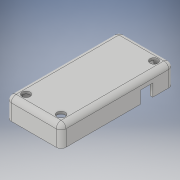
# Autodesk Inventor part: Topcase
Saved by Autodesk Inventor 2019 (Build 230136000, 136)
## iProperties
Created: 2019-05-05
Part Number: Topcase
Material: Generic
Document SubType Name: Modeling
Designer: Henry
Density: 1 g/cm^3
Appearance: Default
Author: Henry
Autodesk Inventor part; units mm, degrees
ref_plane "YZ Plane" through (0, 0, 0) normal (1, 0, 0) x (0, 1, 0)
ref_plane "XZ Plane" through (0, 0, 0) normal (0, 1, 0) x (-1, 0, 0)
ref_plane "XY Plane" through (0, 0, 0) normal (0, 0, 1) x (1, 0, 0)
sketch "Sketch1" plane through (0, 0, 0) normal (0, 1, 0) x (-1, 0, 0)
  line L0 (0, 0) -> (40.5, 0)
  line L1 (40.5, 0) -> (40.5, -87.5)
  line L2 (40.5, -87.5) -> (0, -87.5)
  line L3 (0, -87.5) -> (0, 0)
  dimension "d0" = 40.5
  dimension "d1" = 87.5
  constraints: 8 end point, 2 parallel, 1 horizontal, 1 perpendicular
  measures "d0" distance of L1.end L2.end
  measures "d1" distance of L0.end L1.end
extrude "Extrusion1" add sketch "Sketch1" along normal blind 2
sketch "Sketch4" plane through (0, 2, 0) normal (0, 1, 0) x (1, 0, 0)
  line L0 (0, 0) -> (2, 0)
  line L1 (2, 0) -> (2, 87.5)
  line L2 (2, 87.5) -> (0, 87.5)
  line L3 (0, 87.5) -> (0, 0)
  line L4 (-40.5, 87.5) -> (-40.5, 0) projected
  line L5 (-40.5, 0) -> (-42.5, 0)
  line L6 (-42.5, 0) -> (-42.5, 87.5)
  line L7 (-42.5, 87.5) -> (-40.5, 87.5)
  line L8 (-40.5, 87.5) -> (-40.5, 0)
  line L9 (-42.5, 0) -> (2, 0)
  line L10 (2, 0) -> (2, -2)
  line L11 (2, -2) -> (-42.5, -2)
  line L12 (-42.5, -2) -> (-42.5, 0)
  line L13 (2, 87.5) -> (-42.5, 87.5)
  line L14 (-42.5, 87.5) -> (-42.5, 89.5)
  line L15 (-42.5, 89.5) -> (2, 89.5)
  line L16 (2, 89.5) -> (2, 87.5)
  dimension "d23" = 2
  dimension "d24" = 2
  dimension "d25" = 2
  dimension "d26" = 2
  constraints: 32 end point, 8 parallel, 4 horizontal, 4 perpendicular, 1 point on line
  measures "d23" distance of L2.end L1.end
  measures "d24" distance of L6.end L7.end
  measures "d25" distance of L9.end L10.end
  measures "d26" distance of L13.end L14.end
extrude "Extrusion4" add sketch "Sketch4" against normal blind 17 contours L3 L2 L1 L0 | L0 L10 L11 L12 L5 L9 | L13 L7 L14 L15 L16 L2 | L5 L6 L7 L4
fillet "Fillet1" radius 4 8 edges at (2, -6.5, -89.5) (2, 2, -43.75) (-20.25, 2, -89.5) (-42.5, -6.5, -89.5) (-42.5, 2, -43.75) (-42.5, -6.5, 2) (-20.25, 2, 2) (2, -6.5, 2)
sketch "Sketch5" plane through (0, 0, 0) normal (0, -1, 0) x (1, 0, 0)
  line L0 (-40.5, 0) -> (0, 0) projected
  line L1 (0, 0) -> (-6, 0)
  line L2 (-6, 0) -> (-6, -6)
  line L3 (-6, -6) -> (0, -6)
  line L4 (0, -6) -> (0, 0)
  circle A0 centre (-6, -6) radius 3.35
  line L5 (0, -87.5) -> (-40.5, -87.5) projected
  line L6 (0, -87.5) -> (-6, -87.5)
  line L7 (-6, -87.5) -> (-6, -81.5)
  line L8 (-6, -81.5) -> (0, -81.5)
  line L9 (0, -81.5) -> (0, -87.5)
  circle A1 centre (-6, -81.5) radius 3.25
  line L10 (-40.5, -87.5) -> (-34.5, -87.5)
  line L11 (-40.5, -81.5) -> (-40.5, -87.5)
  line L12 (-40.5, 0) -> (-40.5, -87.5) projected
  line L13 (-40.5, 0) -> (-34.5, 0)
  line L14 (-34.5, 0) -> (-34.5, -6)
  line L15 (-34.5, -6) -> (-40.5, -6)
  line L16 (-40.5, -6) -> (-40.5, 0)
  circle A2 centre (-34.5, -6) radius 3.25
  dimension "d30" = 6
  dimension "d31" = 6
  dimension "d32" = 6.7
  dimension "d33" = 6
  dimension "d34" = 6
  dimension "d35" = 6.5
  dimension "d41" = 6
  dimension "d42" = 6
  dimension "d43" = 6.5
  constraints: 28 end point, 6 parallel, 4 horizontal, 3 centre point, 3 coincident, 3 perpendicular
  measures "d30" distance of L3.end L2.end
  measures "d31" distance of L2.end L1.end
  measures "d32" diameter of A0
  measures "d33" distance of L7.end L8.end
  measures "d34" distance of L6.end L7.end
  measures "d35" diameter of A1
  measures "d41" distance of L14.end L15.end
  measures "d42" distance of L13.end L14.end
  measures "d43" diameter of A2
extrude "Extrusion6" cut sketch "Sketch5" against normal blind 12 contours A2 L15 L14 | L14 L15 A2 | A0 L3 L2 | L2 L3 A0 | A1 L8 L7 | L7 L8 A1
sketch "Sketch6" plane through (0, 0, 0) normal (0, -1, 0) x (1, 0, 0)
  circle A0 centre (-6, -6) radius 3.35 projected
  line L0 (-6, -6) -> (-8.1213, -3.8787) construction
  line L1 (-6, -6) -> (-3, -6) construction
  line L2 (-6, -6) -> (-4.0716, -8.2981) construction
  arc A1 (-2.1433, -10.5963) -> (-10.2426, -1.7574) centre (-6, -6) ccw
  line L3 (-6, -6) -> (-10.2426, -1.7574) construction
  line L4 (-6, -6) -> (0, -6) construction
  line L5 (-6, -6) -> (-2.1433, -10.5963) construction
  circle A2 centre (-6, -81.5) radius 3.25 projected
  arc A3 (-10.2426, -85.7426) -> (-1.4037, -77.6433) centre (-6, -81.5) ccw
  line L6 (-6, -81.5) -> (-10.2426, -85.7426) construction
  line L7 (-6, -81.5) -> (0, -81.5) construction
  line L8 (-6, -81.5) -> (-1.4037, -77.6433) construction
  arc A4 (-8.2981, -83.7981) -> (-3.5104, -79.4109) centre (-6, -81.5) ccw
  line L9 (-3.5104, -79.4109) -> (-1.4037, -77.6433)
  line L10 (-8.2981, -83.7981) -> (-10.2426, -85.7426)
  circle A5 centre (-34.5, -6) radius 3.25 projected
  arc A6 (-28.5, -6) -> (-40.5, -6) centre (-34.5, -6) ccw
  circle A7 centre (-6, -6) radius 3.35 projected
  arc A8 (-3.8467, -8.5662) -> (-8.3688, -3.6312) centre (-6, -6) ccw
  line L11 (-2.1433, -10.5963) -> (-3.8467, -8.5662)
  line L12 (-8.3688, -3.6312) -> (-10.2426, -1.7574)
  arc A9 (-31.25, -6) -> (-37.75, -6) centre (-34.5, -6) ccw
  line L13 (-31.25, -6) -> (-28.5, -6)
  line L14 (-37.75, -6) -> (-40.5, -6)
  point P0 (0, 0)
  dimension "d47" = 135
  dimension "d48" = 175
  dimension "d49" = 6
  dimension "d50" = 135
  dimension "d51" = 175
  dimension "d52" = 6
  dimension "d53" = 135
  dimension "d54" = 175
  dimension "d55" = 3.25
  dimension "d57" = 6
  constraints: 30 end point, 15 point on circle, 6 centre point, 6 coincident, 4 collinear, 4 horizontal, 4 point on line, 3 equal length, 1 horizontal alignment, 1 other
  measures "d47" angle of L1 L0
  measures "d48" angle of L0 L2
  measures "d49" radius of A1
  measures "d50" angle of L4 L3
  measures "d51" angle of L3 L5
  measures "d52" radius of A3
  measures "d53" angle of L6 L7
  measures "d54" angle of L6 L8
  measures "d55" radius of A4
  measures "d57" radius of A6
extrude "Extrusion7" add sketch "Sketch6" along normal blind 14 contours A0 L12 A1 L11 | A2 L9 A3 L10 | A5 L14 A6 L13
sketch "Sketch9" plane through (0, -15, 0) normal (0, -1, 0) x (1, 0, 0)
  line L0 (0, -87.5) -> (0, -81.5) projected
  line L1 (0, -87.5) -> (0, -72.4886)
  line L2 (2, -85.5) -> (2, -2) projected
  line L3 (0, -72.4886) -> (2, -72.4886)
  line L4 (2, -72.4886) -> (2, -62.4886)
  line L5 (2, -62.4886) -> (0, -62.4886)
  line L6 (0, -62.4886) -> (0, -72.4886)
  point P0 (0, 0)
  dimension "d74" = 15.0114
  dimension "d75" = 10
  constraints: 10 end point, 2 parallel, 1 collinear, 1 horizontal, 1 perpendicular, 1 point on line
  measures "d74" distance of L0.start L1.end
  measures "d75" distance of L4.end L3.end
extrude "Extrusion10" cut sketch "Sketch9" against normal blind 10
sketch "Sketch10" plane through (0, -14, 0) normal (0, -1, 0) x (1, 0, 0)
  circle A0 centre (-34.5, -6) radius 3.25 projected
  line L0 (-28.5, -6) -> (-31.25, -6) projected
  line L1 (-37.75, -6) -> (-40.5, -6) projected
  arc A1 (-28.5, -6) -> (-40.5, -6) centre (-34.5, -6) ccw
  arc A2 (-32.5, -6) -> (-36.5, -6) centre (-34.5, -6) ccw
  line L2 (-40.5, -6) -> (-36.5, -6)
  line L3 (-40.5, -87.5) -> (-40.5, 0) projected
  line L4 (-32.5, -6) -> (-28.5, -6)
  arc A3 (-8.3688, -3.6312) -> (-3.8467, -8.5662) centre (-6, -6) ccw projected
  arc A4 (-2.1433, -10.5963) -> (0, -6) centre (-6, -6) ccw projected
  arc A5 (-6, 0) -> (-10.2426, -1.7574) centre (-6, -6) ccw projected
  arc A6 (-2.1433, -10.5963) -> (-10.2426, -1.7574) centre (-6, -6) ccw
  arc A7 (-4.7144, -7.5321) -> (-7.4142, -4.5858) centre (-6, -6) ccw
  line L5 (-6, -6) -> (-4.7144, -7.5321) construction
  line L6 (-6, -6) -> (-4, -6) construction
  line L7 (-10.2426, -1.7574) -> (-8.3688, -3.6312) projected
  line L8 (-7.4142, -4.5858) -> (-10.2426, -1.7574)
  line L9 (-4.7144, -7.5321) -> (-2.1433, -10.5963)
  circle A8 centre (-6, -81.5) radius 3.25 projected
  arc A9 (-10.2426, -85.7426) -> (-6, -87.5) centre (-6, -81.5) ccw projected
  line L10 (-1.4037, -77.6433) -> (-3.5104, -79.4109) projected
  arc A10 (-10.2426, -85.7426) -> (-1.4037, -77.6433) centre (-6, -81.5) ccw
  arc A11 (-7.4142, -82.9142) -> (-4.4679, -80.2144) centre (-6, -81.5) ccw
  line L11 (-4.4679, -80.2144) -> (-1.4037, -77.6433)
  line L12 (-7.4142, -82.9142) -> (-10.2426, -85.7426)
  point P0 (0, 0)
  dimension "d78" = 2
  dimension "d79" = 2
  dimension "d80" = 50
  dimension "d81" = 2
  constraints: 16 end point, 12 point on circle, 6 centre point, 6 coincident, 2 collinear, 1 equal length, 1 horizontal, 1 perpendicular, 1 point on line, 1 other
  measures "d78" radius of A2
  measures "d79" radius of A7
  measures "d80" angle of L5 L6
  measures "d81" radius of A11
extrude "Extrusion11" add sketch "Sketch10" along normal blind 1.4 contours L4 A2 L2 A0 | A0 L1 A1 L0 | L7 A5 A6 A4 L9 A7 L8 | A8 L12 A11 L11 | A8 L10 A10 A9 L12 picked at (-32.5747, -3.948) picked at (-7.6808, -83.7579)
fillet "Fillet4" radius 1.5 3 edges at (-3.5301, -14, -3.7368) (-34.5, -14, -2.75) (-3.8043, -14, -83.8962)
body "Solid1"
